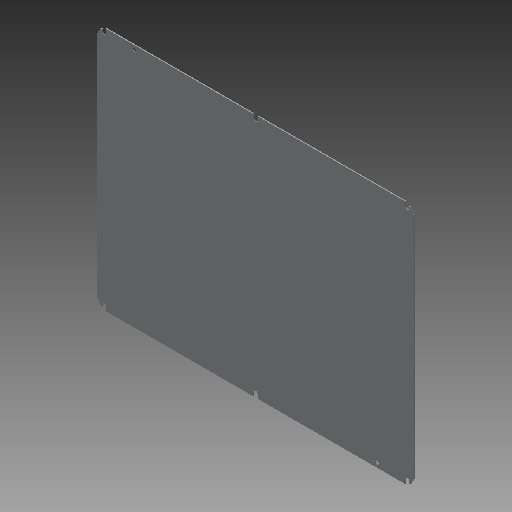
# Autodesk Inventor part: 1100_02_16 (2)
Saved by Autodesk Inventor 2019.3 (Build 233278000, 278)
## iProperties
Category: PARTsolutions
Company: RITTAL
Created: 2018-11-14
Part Number: 1100_02_16 (2)
Material: Generic
Catalog Web Link: www.cadenas.de
Description: Montageplatte AE-Montageplatte AE
Vendor: RITTAL
Document SubType Name: Modeling
Designer: psadmin
Manufacturer: RITTAL
Mass: 2061.02 g
Surface Area: 13845.5 cm^2
Volume: 2061.02 cm^3
Density: 1 g/cm^3
Appearance: PSOLRGB-195-201-196
PSOL_IDENT_0: {$CADENAS_DATA\23d-libs\rittal_usa\schaltschranksys\kompakt_schaltschr\ae\parts_ae\montageplatte_ae.
PSOL_IDENT_1: prj},204 {VTYP=3D},{NB=1100_02_16 (2)},{LINA=1100_02_16 (2)},{NN=Montageplatte AE},{DATE=08.11.2018
PSOL_IDENT_2: 06:46:30},{GEOMDATE=18.08.2014 07:17:00},{VERSION=v140818072938},{LINEID=220},{WBVAR=DETAIL},{WBNUME
PSOL_IDENT_3: RIC=DETAIL}  {NB=1100_02_16 (2)},{LINA=1100_02_16 (2)},{KT=DUMMY},{BEST=1100_02_16},{VERS=3},{DETAIL=
PSOL_IDENT_4: 2},{BEZ1=MIN},{BEZ2=MIN},{BEZ3=MIN},{Q=944.000},{K=730.000},{A=1000.000},{B=760.000},{C=300.000},{D=
PSOL_IDENT_5: 303.000},{E=113.000},{F=70.000},{G=30.000},{H=705.000},{I=667.200},{P=905.000},{R=495.000},{S=755.00
PSOL_IDENT_6: 0},{T=616.400},{U=675.000},{V=27.000},{W=698.000},{X=0.000},{Y=0.000},{B1=1000},{H1=760},{T1=300},{F
PSOL_IDENT_7: 1=944},{G1=730},{S1=3.0},{GEW=56.0}
NN: Montageplatte AE
NT: Montageplatte AE
NB: 1100_02_16 (2)
NBSYN: $BEST. ($DETAIL.)
LINA: 1100_02_16 (2)
BEST: 1100_02_16
VERS: 3
DETAIL: 2
BEZ1: 0
BEZ2: 0
BEZ3: 0
Q: 944
K: 730
A: 1000
B: 760
C: 300
D: 303
E: 113
F: 70
G: 30
H: 705
I: 667.2
P: 905
R: 495
S: 755
T: 616.4
U: 675
V: 27
W: 698
X: 0
Y: 0
B1: 1000
H1: 760
T1: 300
F1: 944
G1: 730
S1: 3
GEW: 56
SUPPLIER: RITTAL
ARTICLENO: 1100_02_16 (2)
BOMINFO: 1100_02_16 (2)
CREATOR: CADENAS GmbH
Title: 1100_02_16 (2)
Author: Cadenas PARTsolutions
Comments: Montageplatte AE
Autodesk Inventor part; units mm, degrees
sketch "Skizze_3" plane through (0, 0, 0) normal (0, 0, 1) x (1, 0, 0)
  line L0 (-472, 11.4545) -> (-462.5, -5)
  line L1 (-462.5, -5) -> (-458.5, -5)
  line L2 (-458.5, -5) -> (-458.5, 0)
  arc A0 (-446.5, 0) -> (-458.5, 0) centre (-452.5, 0) ccw
  line L3 (-446.5, 0) -> (-446.5, -12.5)
  line L4 (-446.5, -12.5) -> (-6, -12.5)
  line L5 (-6, -12.5) -> (-6, 0)
  arc A1 (6, 0) -> (-6, 0) centre (0, 0) ccw
  line L6 (6, 0) -> (6, -12.5)
  line L7 (6, -12.5) -> (446.5, -12.5)
  line L8 (446.5, -12.5) -> (446.5, 0)
  arc A2 (458.5, 0) -> (446.5, 0) centre (452.5, 0) ccw
  line L9 (458.5, 0) -> (458.5, -5)
  line L10 (458.5, -5) -> (462.5, -5)
  line L11 (462.5, -5) -> (472, 11.4545)
  line L12 (472, 11.4545) -> (472, 693.5455)
  line L13 (472, 693.5455) -> (462.5, 710)
  line L14 (462.5, 710) -> (458.5, 710)
  line L15 (458.5, 710) -> (458.5, 705)
  arc A3 (446.5, 705) -> (458.5, 705) centre (452.5, 705) ccw
  line L16 (446.5, 705) -> (446.5, 717.5)
  line L17 (446.5, 717.5) -> (6, 717.5)
  line L18 (6, 717.5) -> (6, 705)
  arc A4 (-6, 705) -> (6, 705) centre (0, 705) ccw
  line L19 (-6, 705) -> (-6, 717.5)
  line L20 (-6, 717.5) -> (-446.5, 717.5)
  line L21 (-446.5, 717.5) -> (-446.5, 705)
  arc A5 (-458.5, 705) -> (-446.5, 705) centre (-452.5, 705) ccw
  line L22 (-458.5, 705) -> (-458.5, 710)
  line L23 (-458.5, 710) -> (-462.5, 710)
  line L24 (-462.5, 710) -> (-472, 693.5455)
  line L25 (-472, 693.5455) -> (-472, 11.4545)
  circle A6 centre (362.5, 0) radius 5
  circle A7 centre (-362.5, 705) radius 5
  constraints: 52 end point, 12 point on circle, 8 centre point
extrude "Extrusion1" add sketch "Skizze_3" against normal blind 3
ref_plane "DPF11_XY" through (472, 352.5, 0) normal (0, 0, 1) x (1, 0, 0)
ref_plane "DPF11_YZ" through (472, 352.5, 0) normal (1, 0, 0) x (0, 1, 0)
ref_plane "DPF11_ZX" through (472, 352.5, 0) normal (0, 1, 0) x (0, 0, 1)
ref_plane "DPF12_XY" through (-472, 352.5, 0) normal (0, 0, 1) x (1, 0, 0)
ref_plane "DPF12_YZ" through (-472, 352.5, 0) normal (1, 0, 0) x (0, 1, 0)
ref_plane "DPF12_ZX" through (-472, 352.5, 0) normal (0, 1, 0) x (0, 0, 1)
ref_plane "DPF21_XY" through (452.5, 705, 0) normal (0, 0, 1) x (1, 0, 0)
ref_plane "DPF21_YZ" through (452.5, 705, 0) normal (1, 0, 0) x (0, 1, 0)
ref_plane "DPF21_ZX" through (452.5, 705, 0) normal (0, 1, 0) x (0, 0, 1)
ref_plane "DPF22_XY" through (-452.5, 705, 0) normal (0, 0, 1) x (1, 0, 0)
ref_plane "DPF22_YZ" through (-452.5, 705, 0) normal (1, 0, 0) x (0, 1, 0)
ref_plane "DPF22_ZX" through (-452.5, 705, 0) normal (0, 1, 0) x (0, 0, 1)
ref_plane "DPG11_XY" through (0, -12.5, 0) normal (0, 0, 1) x (1, 0, 0)
ref_plane "DPG11_YZ" through (0, -12.5, 0) normal (1, 0, 0) x (0, 1, 0)
ref_plane "DPG11_ZX" through (0, -12.5, 0) normal (0, 1, 0) x (0, 0, 1)
ref_plane "DPG12_XY" through (0, 717.5, 0) normal (0, 0, 1) x (1, 0, 0)
ref_plane "DPG12_YZ" through (0, 717.5, 0) normal (1, 0, 0) x (0, 1, 0)
ref_plane "DPG12_ZX" through (0, 717.5, 0) normal (0, 1, 0) x (0, 0, 1)
ref_plane "DPG21_XY" through (452.5, 0, 0) normal (0, 0, 1) x (1, 0, 0)
ref_plane "DPG21_YZ" through (452.5, 0, 0) normal (1, 0, 0) x (0, 1, 0)
ref_plane "DPG21_ZX" through (452.5, 0, 0) normal (0, 1, 0) x (0, 0, 1)
ref_plane "DPG22_XY" through (452.5, 705, 0) normal (0, 0, 1) x (1, 0, 0)
ref_plane "DPG22_YZ" through (452.5, 705, 0) normal (1, 0, 0) x (0, 1, 0)
ref_plane "DPG22_ZX" through (452.5, 705, 0) normal (0, 1, 0) x (0, 0, 1)
ref_plane "montageplatte_XY" through (-452.5, 0, 0) normal (0, 0, 1) x (1, 0, 0)
ref_plane "montageplatte_YZ" through (-452.5, 0, 0) normal (1, 0, 0) x (0, 1, 0)
ref_plane "montageplatte_ZX" through (-452.5, 0, 0) normal (0, 1, 0) x (0, 0, 1)
body "Solid1"
